Autodesk Inventor part; units mm, degrees
(part 2 of 2)
equation "\"Wall_thickness\" = 1"
equation "\"d33\" = 2"
equation "\"Overall_height\" = 10"
equation "\"Hole_height\" = 8.4"
body "Solid2"
